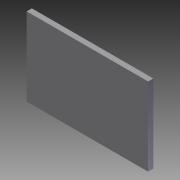
# Autodesk Inventor part: CatcherBox
Saved by Autodesk Inventor 2012 SP2 (Build 160219200, 219)
## iProperties
Created: 2013-07-29
Part Number: CatcherBox
Material: Default
Document SubType Name: Modeling
Designer: 1
Density: 1 g/cm^3
Author: 1
Autodesk Inventor part; units mm, degrees
ref_plane "YZ Plane" through (0, 0, 0) normal (1, 0, 0) x (0, 1, 0)
ref_plane "XZ Plane" through (0, 0, 0) normal (0, 1, 0) x (-1, 0, 0)
ref_plane "XY Plane" through (0, 0, 0) normal (0, 0, 1) x (1, 0, 0)
sketch "Sketch1" plane through (0, 0, 0) normal (0, 0, 1) x (1, 0, 0)
  line L0 (0, 225) -> (0, -225)
  line L1 (0, -225) -> (-700, -225)
  line L2 (-700, -225) -> (-700, 225)
  line L3 (-700, 225) -> (0, 225)
  point P0 (0, 0)
  constraints: 8 end point, 2 horizontal, 2 vertical, 4 other
extrude "Extrusion1" add sketch "Sketch1" along normal blind 30
sketch "Sketch2" plane through (0, 0, 30) normal (0, 0, 1) x (1, 0, 0)
  line L0 (0, -225) -> (-700, -225) projected
  line L1 (0, 225) -> (0, -225) projected
  line L2 (-700, 225) -> (0, 225) projected
  line L3 (-700, -225) -> (-700, 225) projected
  line L4 (-15, 210) -> (-15, -210)
  line L5 (-15, -210) -> (-685, -210)
  line L6 (-685, -210) -> (-685, 210)
  line L7 (-685, 210) -> (-15, 210)
  point P0 (0, 0)
  dimension "d2" = 15
  constraints: 8 end point, 3 other
  measures "d2" distance between parallel lines of L3 L6
extrude "Extrusion2" cut sketch "Sketch2" against normal blind 3 contours L4 L5 L6 L7
sketch "Sketch3" plane through (0, 0, 27) normal (0, 0, 1) x (1, 0, 0)
  line L0 (-15, 210) -> (-685, 210) projected
  line L1 (-685, 210) -> (-685, -210) projected
  line L2 (-685, -210) -> (-15, -210) projected
  line L3 (-525, 210) -> (-525, -210)
  point P0 (0, 0)
  dimension "d5" = 160
  constraints: 2 end point, 2 point on line, 1 perpendicular
  measures "d5" distance between parallel lines of L1 L3
extrude "Extrusion3" cut sketch "Sketch3" against normal blind 23.6375
body "Solid1"
